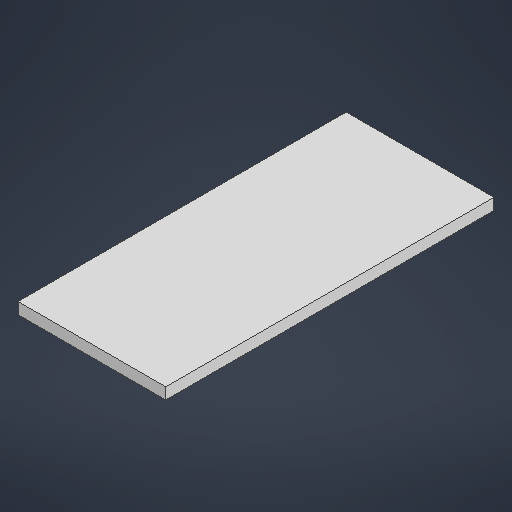
# Autodesk Inventor part: Solor Cleaner - Solor Panal
Saved by Autodesk Inventor 2026 (Build 300175050, 175E)
## iProperties
Created: 2026-02-09
Part Number: Solor Cleaner - Solor Panal
Material: Generic
Document SubType Name: Modeling
Designer: 268021
Density: 1 g/cm^3
Appearance: Default
Author: 268021
Autodesk Inventor part; units mm, degrees
ref_plane "YZ Plane" through (0, 0, 0) normal (1, 0, 0) x (0, 1, 0)
ref_plane "XZ Plane" through (0, 0, 0) normal (0, 1, 0) x (-1, 0, 0)
ref_plane "XY Plane" through (0, 0, 0) normal (0, 0, 1) x (1, 0, 0)
sketch "Sketch1" plane through (0, 0, 0) normal (0, 1, 0) x (-1, 0, 0)
  line L0 (0, 0) -> (-660.4, 0)
  line L1 (-660.4, 0) -> (-660.4, -1466.85)
  line L2 (-660.4, -1466.85) -> (0, -1466.85)
  line L3 (0, -1466.85) -> (0, 0)
  dimension "d0" = 660.4
  dimension "d1" = 1466.85
  constraints: 8 end point, 2 parallel, 1 horizontal, 1 perpendicular
  measures "d0" distance of L2.end L1.end
  measures "d1" distance of L1.end L0.end
extrude "Extrusion1" add sketch "Sketch1" along normal blind 50.8
body "Solid1"
